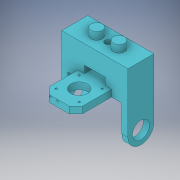
# Autodesk Inventor part: joint1_level_part_2
Saved by Autodesk Inventor 2019 (Build 230136000, 136)
## iProperties
Created: 2019-12-26
Part Number: joint1_level_part_2
Material: Пластик АБС
Document SubType Name: Modeling
Designer: Петров Иван
Density: 1.06 g/cm^3
Appearance: Серо-синий
Author: Петров Иван
Autodesk Inventor part; units mm, degrees
ref_plane "YZ Plane" through (0, 0, 0) normal (1, 0, 0) x (0, 1, 0)
ref_plane "XZ Plane" through (0, 0, 0) normal (0, 1, 0) x (-1, 0, 0)
sketch "Эскиз1" plane through (0, 0, 0) normal (1, 0, 0) x (0, 1, 0)
  line L0 (-6, -6.0208) -> (-6, 6.0208)
  arc A0 (-6, -6.0208) -> (6, -6.0208) centre (0, 0) ccw
  line L1 (6, 6.0208) -> (6, -6.0208)
  arc A1 (6, 6.0208) -> (-6, 6.0208) centre (0, 0) ccw
  circle A2 centre (0, 0) radius 17.5
  line L2 (0, 17.5) -> (80, 17.5)
  line L3 (80, 17.5) -> (80, -17.5)
  line L4 (80, -17.5) -> (0, -17.5)
  line L5 (0, -17.5) -> (0, -8.5)
  line L6 (0, 8.5) -> (0, 17.5)
  dimension "d0" = 35
  dimension "d1" = 80
  constraints: 14 end point, 6 point on circle, 3 parallel, 2 centre point, 1 coincident, 1 horizontal, 1 perpendicular, 1 vertical alignment, 2 other
  measures "d1" distance of L3.end L4.end
extrude "Выдавливание1" add sketch "Эскиз1" along normal blind 45 contours A0 L5 A2 L6 A1 L0 | A0 L1 A1 L6 A2 L5 | A2 L2 L3 L4
sketch "Эскиз2" plane through (45, 0, 0) normal (1, 0, 0) x (0, 0, -1)
  line L0 (17.5, 80) -> (-17.5, 80) projected
  line L1 (17.5, 0) -> (17.5, 80) projected
  line L2 (-17.5, 80) -> (17.5, 80)
  line L3 (17.5, 80) -> (17.5, 57)
  line L4 (17.5, 57) -> (-17.5, 57)
  line L5 (-17.5, 57) -> (-17.5, 80)
  point P0 (0, 0)
  dimension "d4" = 23
  constraints: 8 end point, 2 parallel, 1 horizontal, 1 perpendicular, 1 point on line
  measures "d4" distance of L2.end L3.end
extrude "Выдавливание2" add sketch "Эскиз2" along normal blind 22
ref_plane "РабПлоскость1" through (22.5, 0, 17.5) normal (1, 0, 0) x (0, 0, -1)
mirror "Зеркальное отражение1" about plane through (22.5, 0, 17.5) normal (1, 0, 0) of "Выдавливание2"
sketch "Эскиз3" plane through (45, 0, 0) normal (1, 0, 0) x (0, 0, -1)
  arc A0 (6.0208, -6) -> (6.0208, 6) centre (0, 0) ccw projected
  line L0 (6.0208, -6) -> (-6.0208, -6) projected
  arc A1 (-6.0208, 6) -> (-6.0208, -6) centre (0, 0) ccw projected
  line L1 (6.0208, 6) -> (-6.0208, 6) projected
  line L2 (17.5, 57) -> (-17.5, 57) projected
  line L3 (-17.5, 57) -> (-17.5, 0) projected
  arc A2 (-17.5, 0) -> (17.5, 0) centre (0, 0) ccw projected
  line L4 (17.5, 0) -> (17.5, 57) projected
sketch "Эскиз4" plane through (67, 0, 0) normal (1, 0, 0) x (0, 0, -1)
  arc A0 (6.0208, -6) -> (6.0208, 6) centre (0, 0) ccw
  line L0 (6.0208, -6) -> (-6.0208, -6)
  arc A1 (-6.0208, 6) -> (-6.0208, -6) centre (0, 0) ccw
  line L1 (6.0208, 6) -> (-6.0208, 6)
  line L2 (17.5, 37) -> (-17.5, 37)
  line L3 (-17.5, 37) -> (-17.5, 0)
  arc A2 (-17.5, 0) -> (17.5, 0) centre (0, 0) ccw
  line L4 (17.5, 0) -> (17.5, 37)
  line L5 (17.5, 0) -> (17.5, 57) projected
  line L6 (-17.5, 37) -> (17.5, 37)
  line L7 (17.5, 37) -> (17.5, 57)
  line L8 (17.5, 57) -> (-17.5, 57)
  line L9 (-17.5, 57) -> (-17.5, 37)
  constraints: 18 end point, 6 point on circle, 3 centre point, 2 parallel, 1 horizontal, 1 perpendicular
extrude "Выдавливание3" add sketch "Эскиз4" against normal blind 8
mirror "Зеркальное отражение2" about plane through (22.5, 0, 17.5) normal (1, 0, 0) of "Выдавливание3"
sketch "Эскиз5" plane through (67, 80, 17.5) normal (0, 1, 0) x (1, 0, 0)
  line L0 (-89, 35) -> (-89, 0) projected
  line L1 (-89, 35.1034) -> (-89, 0)
  line L2 (-89, 0) -> (-89, 35.1034)
  line L3 (-89, 35) -> (0, 35) projected
  line L4 (-89, 35) -> (0, 35)
  line L5 (-89, 17.5517) -> (-44.5, 17.5517)
  circle A0 centre (-44.5, 17.5517) radius 4.1
  line L6 (-44.5, 17.5517) -> (-59.5, 17.5517)
  circle A1 centre (-59.5, 17.5517) radius 7.5
  line L7 (-44.5, 17.5517) -> (-29.5, 17.5517)
  circle A2 centre (-29.5, 17.5517) radius 7.5
  point P0 (-67, 17.5)
  dimension "d9" = 8.2
  dimension "d10" = 15
  dimension "d11" = 15
  dimension "d12" = 15
  dimension "d13" = 15
  constraints: 12 end point, 3 centre point, 3 coincident, 3 collinear, 2 horizontal, 1 midpoint, 1 point on line
  measures "d9" diameter of A0
  measures "d10" distance of L6.start L6.end
  measures "d11" diameter of A1
  measures "d12" distance of L6.start L7.end
  measures "d13" diameter of A2
extrude "Выдавливание4" add sketch "Эскиз5" along normal blind 10 contours L5 A1 | L5 A1 | A2
sketch "Эскиз6" plane through (67, 80, 17.5) normal (0, 1, 0) x (1, 0, 0)
  line L0 (-89, 35) -> (-89, 0)
  line L1 (-89, 35.1034) -> (-89, 0)
  line L2 (-89, 0) -> (-89, 35.1034)
  line L3 (-89, 35) -> (0, 35)
  line L4 (-89, 35) -> (0, 35)
  line L5 (-89, 17.5517) -> (-44.5, 17.5517)
  circle A0 centre (-44.5, 17.5517) radius 4.1
  line L6 (-44.5, 17.5517) -> (-59.5, 17.5517)
  circle A1 centre (-59.5, 17.5517) radius 7.5
  line L7 (-44.5, 17.5517) -> (-29.5, 17.5517)
  circle A2 centre (-29.5, 17.5517) radius 7.5
  point P0 (-67, 17.5)
  point P1 (-67, 17.5)
  dimension "d16" = 8.2
  dimension "d17" = 15
  dimension "d18" = 15
  dimension "d19" = 15
  dimension "d20" = 15
  constraints: 16 end point, 3 centre point, 3 coincident, 3 collinear, 2 horizontal, 1 midpoint, 1 point on line
  measures "d16" diameter of A0
  measures "d17" distance of L6.start L6.end
  measures "d18" diameter of A1
  measures "d19" distance of L6.start L7.end
  measures "d20" diameter of A2
extrude "Выдавливание5" cut sketch "Эскиз6" against normal blind 35 contours A0 L7 L5 | L5 L7 A0
sketch "Эскиз7" plane through (0, 0, 17.5) normal (0, 0, 1) x (1, 0, 0)
  line L0 (18.4, 80) -> (18.4, 45) projected
  line L1 (26.6, 80) -> (26.6, 45) projected
  line L2 (0, 57) -> (0, 0) projected
  line L3 (45, 0) -> (0, 0) projected
  line L4 (45, 57) -> (45, 0) projected
  line L5 (45, 57) -> (59, 57) projected
  line L6 (67, 80) -> (67, 0) projected
  line L7 (-22, 80) -> (67, 80) projected
  line L8 (-22, 80) -> (-22, 0) projected
  line L9 (0, 57) -> (-14, 57) projected
  line L10 (18.4, 45) -> (26.6, 45) projected
  line L11 (18.4, 45) -> (8.4, 45)
  line L12 (8.4, 45) -> (8.4, 55)
  line L13 (8.4, 55) -> (36.6, 55)
  line L14 (36.6, 55) -> (36.6, 45)
  line L15 (26.6, 45) -> (36.6, 45)
  line L16 (18.4, 45) -> (26.6, 45)
  line L17 (59, 0) -> (59, 57) projected
  line L18 (67, 0) -> (59, 0) projected
  line L19 (-22, 0) -> (-14, 0) projected
  line L20 (-14, 0) -> (-14, 57) projected
  dimension "d23" = 10
  dimension "d24" = 10
  dimension "d25" = 28.2
  dimension "d26" = 10
  constraints: 12 end point, 4 perpendicular, 1 collinear, 1 horizontal, 1 point on line
  measures "d23" distance of L0.end L11.end
  measures "d24" distance of L11.end L12.end
  measures "d25" distance of L12.end L13.end
  measures "d26" distance of L1.end L14.end
extrude "Выдавливание6" cut sketch "Эскиз7" against normal blind 84.5 contours L13 L1 L10 L0 | L0 L11 L12 L13 | L13 L14 L15 L1
sketch "Эскиз8" plane through (0, 0, 17.5) normal (0, 0, 1) x (1, 0, 0)
  line L0 (8.4, 45) -> (36.6, 45) projected
  line L1 (8.4, 45) -> (0, 45)
  line L2 (0, 45) -> (0, 36)
  line L3 (0, 0) -> (0, 57) projected
  line L4 (45, -17.5) -> (45, 0) projected
  line L5 (0, 36) -> (45, 36)
  line L6 (45, 36) -> (45, -17.5)
  line L7 (45, -17.5) -> (0, -17.5)
  line L8 (0, -17.5) -> (0, 36)
  dimension "d29" = 9
  constraints: 12 end point, 2 horizontal, 2 parallel, 1 perpendicular, 1 point on line
  measures "d29" distance of L1.end L2.end
extrude "Выдавливание7" cut sketch "Эскиз8" against normal blind 85.25
sketch "Эскиз9" plane through (67, 0, 0) normal (1, 0, 0) x (0, 0, -1)
  circle A0 centre (0, 0) radius 11.4
  dimension "d32" = 22.8
  constraints: 1 centre point, 1 coincident
  measures "d32" diameter of A0
extrude "Выдавливание8" cut sketch "Эскиз9" against normal blind 144.5
sketch "Эскиз10" plane through (-22, 80, 17.5) normal (0, 0, 1) x (1, 0, 0)
  line L0 (22, -23) -> (22, -44) projected
  line L1 (67, -23) -> (67, -44) projected
  line L2 (22, -44) -> (67, -44)
  line L3 (67, -44) -> (67, -35)
  line L4 (67, -35) -> (22, -35)
  line L5 (22, -35) -> (22, -44)
  point P0 (22, -80)
  dimension "d35" = 9
  constraints: 8 end point, 2 parallel, 1 horizontal, 1 perpendicular, 1 point on line
  measures "d35" distance of L3.end L2.end
extrude "Выдавливание9" add sketch "Эскиз10" along normal blind 45
sketch "Эскиз11" plane through (67, 45, 17.5) normal (0, 1, 0) x (1, 0, 0)
  line L0 (-67, 0) -> (-67, 35) projected
  line L1 (-67, 0) -> (-44.5, 0)
  line L2 (-67, 0) -> (-58.6, 0) projected
  line L3 (-22, -45) -> (-67, -45) projected
  line L4 (-44.5, -45) -> (-44.5, -21)
  line L5 (-27, -42) -> (-23.5, -38.5)
  line L6 (-23.5, -38.5) -> (-23.5, -3.5)
  line L7 (-23.5, -3.5) -> (-27, 0)
  line L8 (-27, 0) -> (-62, 0)
  line L9 (-62, 0) -> (-65.5, -3.5)
  line L10 (-65.5, -3.5) -> (-65.5, -38.5)
  line L11 (-65.5, -38.5) -> (-62, -42)
  line L12 (-62, -42) -> (-27, -42)
  circle A0 centre (-44.5, -21) radius 11.3
  circle A1 centre (-29, -5.5) radius 1.25
  circle A2 centre (-60, -5.5) radius 1.25
  circle A3 centre (-60, -36.5) radius 1.25
  circle A4 centre (-29, -36.5) radius 1.25
  line L13 (-52.5, -48) -> (-50.5, -48)
  line L14 (-50.5, -41.8) -> (-50.5, -48)
  line L15 (-57.9172, -41.8) -> (-50.5, -41.8)
  line L16 (-65.3, -34.4172) -> (-57.9172, -41.8)
  line L17 (-65.3, -7.5828) -> (-65.3, -34.4172)
  line L18 (-57.9172, -0.2) -> (-65.3, -7.5828)
  line L19 (-31.0828, -0.2) -> (-57.9172, -0.2)
  line L20 (-23.7, -7.5828) -> (-31.0828, -0.2)
  line L21 (-23.7, -34.4172) -> (-23.7, -7.5828)
  line L22 (-31.0828, -41.8) -> (-23.7, -34.4172)
  line L23 (-38.5, -41.8) -> (-31.0828, -41.8)
  line L24 (-38.5, -41.8) -> (-38.5, -48)
  line L25 (-38.5, -48) -> (-36.5, -48)
  line L26 (-36.5, -48) -> (-36.5, -42)
  line L27 (-36.5, -42) -> (-27, -42)
  line L28 (-27, -42) -> (-23.5, -38.5)
  line L29 (-23.5, -38.5) -> (-23.5, -3.5)
  line L30 (-23.5, -3.5) -> (-27, 0)
  line L31 (-27, 0) -> (-62, 0)
  line L32 (-62, 0) -> (-65.5, -3.5)
  line L33 (-65.5, -3.5) -> (-65.5, -38.5)
  line L34 (-65.5, -38.5) -> (-62, -42)
  line L35 (-62, -42) -> (-52.5, -42)
  line L36 (-52.5, -42) -> (-52.5, -48)
  point P0 (-67, 17.5)
  dimension "d38" = 22.5
  dimension "d39" = 24
  constraints: 68 end point, 5 centre point, 1 collinear, 1 midpoint, 1 vertical
  measures "d38" distance of L0.start L1.end
  measures "d39" distance of L4.start L4.end
extrude "Выдавливание10" cut sketch "Эскиз11" against normal blind 45 contours A0 | A1 | A2 | A3 | A4
chamfer "Фаска1" distance 2 angle 45 4 edges at (5.75, 36, 54) (5.75, 36, 23) (36.75, 36, 23) (36.75, 36, 54)
chamfer "Фаска2" distance 6 angle 45 2 edges at (0, 40.5, 62.5) (45, 40.5, 62.5)
sketch "Эскиз13" plane through (-22, 80, 17.5) normal (0, 0, 1) x (1, 0, 0)
  line L0 (81, -80) -> (81, -23) projected
  line L1 (22, -23) -> (8, -23) projected
  line L2 (81, -44) -> (8, -44)
  line L3 (8, -44) -> (8, -23)
  line L4 (8, -23) -> (81, -23)
  line L5 (81, -23) -> (81, -44)
  line L6 (61, -44) -> (67, -44) projected
  line L7 (22, -35) -> (30.4, -35) projected
  line L8 (30.4, -25) -> (58.6, -25) projected
  line L9 (30.4, -35) -> (58.6, -35)
  line L10 (58.6, -35) -> (58.6, -25)
  line L11 (58.6, -25) -> (30.4, -25)
  line L12 (30.4, -25) -> (30.4, -35)
  point P0 (22, -80)
  dimension "d51" = 0
  constraints: 16 end point, 4 parallel, 2 horizontal, 2 perpendicular, 1 point on line
  measures "d51" distance between parallel lines of L6 L2
extrude "Выдавливание12" add sketch "Эскиз13" against normal up to surface (35 mm away)
sketch "Эскиз14" plane through (-22, 80, 62.5) normal (0, 0, 1) x (1, 0, 0)
  line L0 (27.8074, -44.5836) -> (28.32, -44.5836)
  line L1 (28.32, -44.5836) -> (28.4117, -43.1496)
  arc A0 (32.6031, -43.1496) -> (28.4117, -43.1496) centre (30.5074, -43.2836) ccw
  line L2 (32.6031, -43.1496) -> (32.6948, -44.5836)
  line L3 (32.6948, -44.5836) -> (36.9831, -44.5836)
  arc A1 (36.9831, -44.5836) -> (37.0538, -44.5543) centre (36.9831, -44.4836) ccw
  line L4 (37.0538, -44.5543) -> (37.3781, -44.23)
  arc A2 (37.7316, -44.0836) -> (37.3781, -44.23) centre (37.7316, -44.5836) ccw
  line L5 (37.7316, -44.0836) -> (47.4074, -44.0836)
  arc A3 (47.4074, -44.0836) -> (47.5074, -43.9836) centre (47.4074, -43.9836) ccw
  line L6 (47.5074, -43.9836) -> (47.5074, -34.8336)
  arc A4 (47.5074, -34.8336) -> (47.4074, -34.7336) centre (47.4074, -34.8336) ccw
  line L7 (47.4074, -34.7336) -> (44.4816, -34.7336)
  arc A5 (44.1281, -34.5871) -> (44.4816, -34.7336) centre (44.4816, -34.2336) ccw
  line L8 (44.1281, -34.5871) -> (43.8038, -34.2629)
  arc A6 (43.8038, -34.2629) -> (43.7331, -34.2336) centre (43.7331, -34.3336) ccw
  line L9 (43.7331, -34.2336) -> (40.9816, -34.2336)
  arc A7 (40.9816, -34.2336) -> (40.9109, -34.2629) centre (40.9816, -34.3336) ccw
  line L10 (40.9109, -34.2629) -> (40.5867, -34.5871)
  arc A8 (40.2331, -34.7336) -> (40.5867, -34.5871) centre (40.2331, -34.2336) ccw
  line L11 (40.2331, -34.7336) -> (34.9816, -34.7336)
  arc A9 (34.6281, -34.5871) -> (34.9816, -34.7336) centre (34.9816, -34.2336) ccw
  line L12 (34.6281, -34.5871) -> (34.3038, -34.2629)
  arc A10 (34.3038, -34.2629) -> (34.2331, -34.2336) centre (34.2331, -34.3336) ccw
  line L13 (34.2331, -34.2336) -> (31.4816, -34.2336)
  arc A11 (31.4816, -34.2336) -> (31.4109, -34.2629) centre (31.4816, -34.3336) ccw
  line L14 (31.4109, -34.2629) -> (31.0867, -34.5871)
  arc A12 (30.7331, -34.7336) -> (31.0867, -34.5871) centre (30.7331, -34.2336) ccw
  line L15 (30.7331, -34.7336) -> (27.8074, -34.7336)
  arc A13 (27.8074, -34.7336) -> (27.7074, -34.8336) centre (27.8074, -34.8336) ccw
  line L16 (27.7074, -34.8336) -> (27.7074, -44.4836)
  arc A14 (27.7074, -44.4836) -> (27.8074, -44.5836) centre (27.8074, -44.4836) ccw
  circle A15 centre (32.8574, -36.7836) radius 1.25
  circle A16 centre (42.3574, -36.7836) radius 1.25
  line L17 (43.5307, -39.0336) -> (42.914, -40.3336)
  line L18 (42.914, -40.3336) -> (42.8974, -40.3336)
  line L19 (42.8974, -40.3336) -> (42.2974, -39.0336)
  line L20 (42.2974, -39.0336) -> (42.4242, -39.0336)
  line L21 (42.4242, -39.0336) -> (42.6164, -39.4502)
  line L22 (42.6164, -39.4502) -> (43.2057, -39.4502)
  line L23 (43.2057, -39.4502) -> (43.4034, -39.0336)
  line L24 (43.4034, -39.0336) -> (43.5307, -39.0336)
  spline S0 degree 3 poles (40.7107, -39.97) (40.711, -39.9789) (40.7114, -39.9964) (40.7155, -40.022) (40.7217, -40.0467) (40.7306, -40.0706) (40.7424, -40.0934) (40.7567, -40.1152) (40.7731, -40.1363) (40.7922, -40.156) (40.8132, -40.1741) (40.8353, -40.1901) (40.8587, -40.2035) (40.8833, -40.2145) (40.909, -40.2231) (40.9359, -40.2291) (40.9639, -40.2328) (40.983, -40.2333) (40.9927, -40.2336) knots 0 0 0 0 0.061965 0.122122 0.180988 0.239933 0.299906 0.359989 0.421776 0.486576 0.551535 0.615018 0.677259 0.73973 0.80305 0.866495 0.931973 1 1 1 1
  spline S1 degree 3 poles (40.9927, -40.2336) (41.0029, -40.2333) (41.0229, -40.2328) (41.0522, -40.2291) (41.0802, -40.2228) (41.1068, -40.2142) (41.1323, -40.2033) (41.1564, -40.1897) (41.1791, -40.1734) (41.2004, -40.155) (41.22, -40.1344) (41.2373, -40.1115) (41.2523, -40.0867) (41.2655, -40.06) (41.2762, -40.0312) (41.2843, -40.0004) (41.2908, -39.9677) (41.2929, -39.9451) (41.294, -39.9336) knots 0 0 0 0 0.064439 0.126547 0.186887 0.245878 0.304041 0.362191 0.420976 0.48066 0.5406 0.600689 0.661936 0.724443 0.789038 0.856314 0.926352 1 1 1 1
  line L25 (41.294, -39.9336) -> (41.4107, -39.9336)
  spline S2 degree 3 poles (41.4107, -39.9336) (41.41, -39.949) (41.4085, -39.9794) (41.4015, -40.0238) (41.3915, -40.0661) (41.3773, -40.1062) (41.3597, -40.1443) (41.3387, -40.1803) (41.3137, -40.2141) (41.2854, -40.2454) (41.2547, -40.2741) (41.2215, -40.2988) (41.1866, -40.3197) (41.1502, -40.3372) (41.1118, -40.3504) (41.0717, -40.3601) (41.0298, -40.366) (41.0013, -40.3666) (40.9868, -40.3669) knots 0 0 0 0 0.068791 0.135103 0.198979 0.261904 0.323495 0.385195 0.446969 0.509765 0.572251 0.633405 0.693251 0.752583 0.812579 0.873275 0.93555 1 1 1 1
  spline S3 degree 3 poles (40.9868, -40.3669) (40.9725, -40.3666) (40.9445, -40.3659) (40.9036, -40.3603) (40.8647, -40.3515) (40.8278, -40.3391) (40.7933, -40.3225) (40.7608, -40.3025) (40.73, -40.2794) (40.7023, -40.2522) (40.6769, -40.2231) (40.6549, -40.1921) (40.6361, -40.1601) (40.6204, -40.1268) (40.6089, -40.0919) (40.6001, -40.056) (40.5952, -40.0186) (40.5944, -39.9933) (40.594, -39.9804) knots 0 0 0 0 0.069475 0.136517 0.200789 0.26383 0.325735 0.387291 0.449509 0.512968 0.576275 0.63758 0.697903 0.757172 0.816599 0.876653 0.93729 1 1 1 1
  spline S4 degree 3 poles (40.594, -39.9804) (40.5947, -39.9623) (40.5959, -39.9264) (40.6066, -39.8737) (40.6232, -39.8226) (40.6433, -39.7815) (40.6635, -39.7483) (40.6818, -39.721) (40.7031, -39.6916) (40.7279, -39.6603) (40.7556, -39.6266) (40.7864, -39.5908) (40.8206, -39.5531) (40.8446, -39.5274) (40.8571, -39.514) knots 0 0 0 0 0.098702 0.195672 0.292422 0.391343 0.444462 0.504229 0.570352 0.642546 0.722288 0.807921 0.90047 1 1 1 1
  line L26 (40.8571, -39.514) -> (41.1823, -39.1669)
  line L27 (41.1823, -39.1669) -> (40.5774, -39.1669)
  line L28 (40.5774, -39.1669) -> (40.5774, -39.0336)
  line L29 (40.5774, -39.0336) -> (41.4607, -39.0336)
  line L30 (41.4607, -39.0336) -> (40.9565, -39.5716)
  spline S5 degree 3 poles (40.9565, -39.5716) (40.9443, -39.5844) (40.9207, -39.609) (40.8873, -39.6449) (40.8574, -39.6783) (40.8306, -39.709) (40.8077, -39.7374) (40.7873, -39.7628) (40.771, -39.7861) (40.7532, -39.8131) (40.7361, -39.8461) (40.7213, -39.8864) (40.7123, -39.9279) (40.7113, -39.9559) (40.7107, -39.97) knots 0 0 0 0 0.110803 0.212829 0.306101 0.390647 0.466924 0.534481 0.593587 0.644557 0.7362 0.825024 0.911986 1 1 1 1
  line L31 (40.2007, -39.6836) -> (40.0674, -40.3336)
  line L32 (40.0674, -40.3336) -> (39.534, -40.3336)
  line L33 (39.534, -40.3336) -> (39.534, -40.2002)
  line L34 (39.534, -40.2002) -> (39.9762, -40.2002)
  line L35 (39.9762, -40.2002) -> (40.0463, -39.8583)
  spline S6 degree 3 poles (40.0463, -39.8583) (40.0325, -39.8621) (40.0059, -39.8695) (39.9665, -39.8776) (39.9291, -39.8826) (39.9049, -39.8832) (39.8932, -39.8836) knots 0 0 0 0 0.275068 0.532901 0.773973 1 1 1 1
  spline S7 degree 3 poles (39.8932, -39.8836) (39.8786, -39.8833) (39.8501, -39.8826) (39.8083, -39.8767) (39.7685, -39.8674) (39.7306, -39.8543) (39.6946, -39.8376) (39.6609, -39.8168) (39.6289, -39.7925) (39.5992, -39.7645) (39.5722, -39.7337) (39.5486, -39.7006) (39.5284, -39.6655) (39.5123, -39.628) (39.4993, -39.5887) (39.4907, -39.547) (39.485, -39.5033) (39.4844, -39.4735) (39.484, -39.4583) knots 0 0 0 0 0.065808 0.129394 0.190894 0.251281 0.310815 0.370371 0.430768 0.492881 0.555104 0.616067 0.677256 0.73826 0.800762 0.864778 0.931045 1 1 1 1
  spline S8 degree 3 poles (39.484, -39.4583) (39.4843, -39.4477) (39.4848, -39.4267) (39.4873, -39.3954) (39.4921, -39.3648) (39.4985, -39.3349) (39.5069, -39.3057) (39.517, -39.2771) (39.5295, -39.2493) (39.5431, -39.2221) (39.5584, -39.196) (39.5754, -39.1716) (39.5933, -39.1485) (39.6127, -39.1271) (39.6335, -39.1073) (39.6557, -39.0891) (39.679, -39.0722) (39.7038, -39.0573) (39.7294, -39.0436) (39.7564, -39.0323) (39.7841, -39.0222) (39.8128, -39.0142) (39.8426, -39.0079) (39.8734, -39.0036) (39.9051, -39.0005) (39.9266, -39.0003) (39.9374, -39.0002) knots 0 0 0 0 0.044014 0.087434 0.130118 0.172554 0.214555 0.256298 0.298438 0.340849 0.382715 0.423924 0.464246 0.504074 0.543862 0.583567 0.623094 0.663229 0.703551 0.743938 0.784541 0.82575 0.867757 0.910745 0.954914 1 1 1 1
  spline S9 degree 3 poles (39.9374, -39.0002) (39.9504, -39.0005) (39.9759, -39.001) (40.0132, -39.0063) (40.0491, -39.0138) (40.0834, -39.0252) (40.1162, -39.0395) (40.1472, -39.0575) (40.1771, -39.0779) (40.2048, -39.102) (40.2305, -39.1284) (40.2535, -39.1569) (40.2739, -39.1873) (40.2916, -39.2196) (40.3066, -39.2537) (40.3184, -39.2898) (40.328, -39.3276) (40.332, -39.3537) (40.334, -39.3669) knots 0 0 0 0 0.065421 0.128708 0.190236 0.250724 0.310637 0.370766 0.431615 0.493523 0.555883 0.617342 0.678668 0.740711 0.802985 0.866803 0.932347 1 1 1 1
  line L36 (40.334, -39.3669) -> (40.2174, -39.3669)
  spline S10 degree 3 poles (40.2174, -39.3669) (40.2145, -39.3545) (40.209, -39.3307) (40.1969, -39.2972) (40.1821, -39.2674) (40.1645, -39.2408) (40.1435, -39.2176) (40.1195, -39.1969) (40.0926, -39.1783) (40.0628, -39.1628) (40.0313, -39.1495) (39.9983, -39.1407) (39.9647, -39.1345) (39.9421, -39.1339) (39.9307, -39.1336) knots 0 0 0 0 0.094687 0.181994 0.264377 0.34218 0.418618 0.496509 0.577369 0.661511 0.746733 0.831258 0.915206 1 1 1 1
  spline S11 degree 3 poles (39.9307, -39.1336) (39.9195, -39.1339) (39.8976, -39.1345) (39.8654, -39.1391) (39.8343, -39.1462) (39.8045, -39.1569) (39.7757, -39.1698) (39.7486, -39.1864) (39.7222, -39.2055) (39.6975, -39.2274) (39.6749, -39.2516) (39.655, -39.2774) (39.6384, -39.3049) (39.6243, -39.3337) (39.6137, -39.364) (39.6061, -39.3958) (39.6016, -39.429) (39.601, -39.4517) (39.6007, -39.4633) knots 0 0 0 0 0.064207 0.126425 0.18768 0.248216 0.308305 0.369661 0.431699 0.495947 0.559758 0.622295 0.683911 0.745092 0.80674 0.869087 0.93329 1 1 1 1
  spline S12 degree 3 poles (39.6007, -39.4633) (39.601, -39.4737) (39.6014, -39.4941) (39.6054, -39.524) (39.6122, -39.5522) (39.6216, -39.579) (39.6336, -39.6043) (39.6482, -39.6283) (39.6658, -39.6504) (39.6859, -39.6709) (39.7079, -39.6898) (39.7322, -39.7059) (39.7583, -39.7194) (39.7859, -39.7311) (39.8156, -39.7395) (39.8468, -39.7458) (39.88, -39.7495) (39.9026, -39.75) (39.9143, -39.7502) knots 0 0 0 0 0.065351 0.127916 0.18836 0.247216 0.30563 0.36377 0.422661 0.482687 0.5433 0.604118 0.664965 0.727413 0.791468 0.858055 0.927037 1 1 1 1
  spline S13 degree 3 poles (39.9143, -39.7502) (39.9243, -39.75) (39.9451, -39.7496) (39.9771, -39.7463) (40.0106, -39.741) (40.0456, -39.7337) (40.0823, -39.7242) (40.1204, -39.7128) (40.1602, -39.6992) (40.1869, -39.6889) (40.2007, -39.6836) knots 0 0 0 0 0.102203 0.211023 0.3251 0.446502 0.573788 0.708901 0.850358 1 1 1 1
  line L37 (36.754, -39.0336) -> (36.1374, -40.3336)
  line L38 (36.1374, -40.3336) -> (36.1207, -40.3336)
  line L39 (36.1207, -40.3336) -> (35.5207, -39.0336)
  line L40 (35.5207, -39.0336) -> (35.6475, -39.0336)
  line L41 (35.6475, -39.0336) -> (35.8397, -39.4502)
  line L42 (35.8397, -39.4502) -> (36.429, -39.4502)
  line L43 (36.429, -39.4502) -> (36.6267, -39.0336)
  line L44 (36.6267, -39.0336) -> (36.754, -39.0336)
  spline S14 degree 3 poles (35.244, -39.6911) (35.2435, -39.7145) (35.2423, -39.7605) (35.2327, -39.828) (35.2171, -39.8927) (35.1951, -39.9544) (35.1671, -40.0135) (35.1326, -40.0696) (35.0918, -40.1229) (35.0452, -40.1727) (34.9941, -40.2182) (34.9394, -40.2582) (34.8812, -40.2915) (34.8201, -40.3194) (34.7556, -40.3408) (34.688, -40.3558) (34.6173, -40.3651) (34.5691, -40.3663) (34.5446, -40.3669) knots 0 0 0 0 0.064558 0.127014 0.187955 0.248014 0.307748 0.368235 0.42947 0.492743 0.556258 0.618217 0.679655 0.741246 0.803415 0.866815 0.932328 1 1 1 1
  spline S15 degree 3 poles (34.5446, -40.3669) (34.5296, -40.3667) (34.5001, -40.3664) (34.4563, -40.3629) (34.4137, -40.3571) (34.3723, -40.3493) (34.3318, -40.3396) (34.2925, -40.3269) (34.2542, -40.3124) (34.2171, -40.2957) (34.1815, -40.2769) (34.1473, -40.2564) (34.1148, -40.234) (34.0838, -40.21) (34.0548, -40.1838) (34.0269, -40.1562) (34.0012, -40.1265) (33.9853, -40.1055) (33.9774, -40.095) knots 0 0 0 0 0.068548 0.135683 0.201215 0.265682 0.329267 0.392395 0.45507 0.517127 0.57879 0.63974 0.700192 0.759806 0.819628 0.879355 0.939512 1 1 1 1
  line L45 (33.9774, -40.095) -> (34.0795, -40.0169)
  spline S16 degree 3 poles (34.0795, -40.0169) (34.0867, -40.0256) (34.1012, -40.0428) (34.1245, -40.067) (34.1487, -40.0897) (34.174, -40.111) (34.2006, -40.1301) (34.2281, -40.148) (34.2567, -40.1641) (34.2964, -40.1836) (34.3483, -40.2039) (34.4135, -40.2209) (34.4817, -40.2318) (34.5282, -40.233) (34.5519, -40.2336) knots 0 0 0 0 0.063163 0.125475 0.187121 0.248294 0.309295 0.36985 0.430973 0.492456 0.616148 0.740844 0.868183 1 1 1 1
  spline S17 degree 3 poles (34.5519, -40.2336) (34.5649, -40.2334) (34.5908, -40.2331) (34.6293, -40.2292) (34.6671, -40.2236) (34.7041, -40.2154) (34.7404, -40.205) (34.7761, -40.1926) (34.8107, -40.1773) (34.8447, -40.1603) (34.8773, -40.1411) (34.9082, -40.1202) (34.9372, -40.0978) (34.9643, -40.0738) (34.9896, -40.0483) (35.0129, -40.021) (35.0342, -39.9921) (35.0538, -39.9619) (35.0713, -39.9305) (35.086, -39.8978) (35.099, -39.8643) (35.1093, -39.8297) (35.1174, -39.7942) (35.123, -39.7577) (35.1269, -39.7204) (35.1272, -39.695) (35.1274, -39.6823) knots 0 0 0 0 0.043955 0.087502 0.130463 0.172752 0.215403 0.25765 0.300153 0.343121 0.385925 0.427686 0.468818 0.509492 0.549883 0.58998 0.630405 0.670869 0.711384 0.751627 0.791776 0.832459 0.873319 0.914543 0.956924 1 1 1 1
  spline S18 degree 3 poles (35.1274, -39.6823) (35.1269, -39.6631) (35.126, -39.6253) (35.1178, -39.5701) (35.1054, -39.5171) (35.0867, -39.4668) (35.0637, -39.4186) (35.0346, -39.3732) (35.001, -39.33) (34.9623, -39.2899) (34.9198, -39.2533) (34.8742, -39.2211) (34.8256, -39.1942) (34.7746, -39.1719) (34.7207, -39.1547) (34.6641, -39.1426) (34.6049, -39.1347) (34.5644, -39.134) (34.5438, -39.1336) knots 0 0 0 0 0.064323 0.12629 0.186726 0.246146 0.305576 0.365429 0.426326 0.48884 0.551725 0.613919 0.675484 0.737334 0.800229 0.864502 0.931041 1 1 1 1
  spline S19 degree 3 poles (34.5438, -39.1336) (34.5211, -39.1342) (34.4764, -39.1354) (34.4109, -39.1459) (34.3482, -39.1628) (34.2883, -39.1866) (34.2313, -39.2174) (34.1773, -39.2548) (34.126, -39.2991) (34.0952, -39.333) (34.0795, -39.3502) knots 0 0 0 0 0.128515 0.252949 0.374755 0.49594 0.617181 0.740909 0.867811 1 1 1 1
  line L46 (34.0795, -39.3502) -> (33.9774, -39.2729)
  spline S20 degree 3 poles (33.9774, -39.2729) (33.9856, -39.2623) (34.002, -39.2411) (34.0285, -39.2113) (34.0565, -39.1833) (34.0861, -39.1572) (34.1169, -39.1327) (34.1497, -39.1103) (34.1838, -39.0897) (34.2192, -39.0709) (34.2559, -39.0542) (34.2938, -39.04) (34.3327, -39.0277) (34.3727, -39.0175) (34.4138, -39.0096) (34.4559, -39.0043) (34.4991, -39.0007) (34.5282, -39.0004) (34.543, -39.0002) knots 0 0 0 0 0.061674 0.123053 0.183475 0.243727 0.304279 0.364863 0.425946 0.487391 0.54922 0.611144 0.673529 0.736961 0.800785 0.866013 0.932101 1 1 1 1
  spline S21 degree 3 poles (34.543, -39.0002) (34.557, -39.0003) (34.5846, -39.0005) (34.6255, -39.0036) (34.6652, -39.0079) (34.7037, -39.0143) (34.7413, -39.0219) (34.7775, -39.032) (34.8128, -39.0433) (34.847, -39.0567) (34.88, -39.0717) (34.9119, -39.0887) (34.9426, -39.1075) (34.9724, -39.1278) (35.0009, -39.1501) (35.0282, -39.1741) (35.0546, -39.1998) (35.071, -39.2183) (35.0792, -39.2276) knots 0 0 0 0 0.069663 0.13775 0.203917 0.26878 0.332414 0.394754 0.45618 0.516996 0.577396 0.637198 0.696999 0.756756 0.816554 0.876948 0.938132 1 1 1 1
  spline S22 degree 3 poles (35.0792, -39.2276) (35.0924, -39.2438) (35.1185, -39.2759) (35.152, -39.328) (35.1807, -39.3824) (35.2038, -39.4394) (35.2219, -39.4988) (35.2345, -39.5608) (35.2426, -39.6251) (35.2436, -39.6689) (35.244, -39.6911) knots 0 0 0 0 0.124329 0.247156 0.36878 0.490734 0.613614 0.738958 0.867311 1 1 1 1
  line L47 (32.1714, -40.2836) -> (32.3842, -40.2836)
  line L48 (32.5718, -39.1836) -> (32.1714, -40.2836)
  line L49 (32.0718, -39.1836) -> (32.5718, -39.1836)
  line L50 (31.6714, -40.2836) -> (32.0718, -39.1836)
  line L51 (31.4585, -40.2836) -> (31.6714, -40.2836)
  line L52 (31.8589, -39.1836) -> (31.4585, -40.2836)
  line L53 (31.6589, -39.1836) -> (31.8589, -39.1836)
  line L54 (31.7317, -38.9836) -> (31.6589, -39.1836)
  line L55 (32.8574, -38.9836) -> (31.7317, -38.9836)
  line L56 (32.3842, -40.2836) -> (32.8574, -38.9836)
  line L57 (37.5474, -39.0336) -> (37.564, -39.0336)
  line L58 (37.564, -39.0336) -> (38.114, -40.3336)
  line L59 (38.114, -40.3336) -> (37.989, -40.3336)
  line L60 (37.989, -40.3336) -> (37.5557, -39.3091)
  line L61 (37.5557, -39.3091) -> (37.1224, -40.3336)
  line L62 (37.1224, -40.3336) -> (36.9974, -40.3336)
  line L63 (36.9974, -40.3336) -> (37.5474, -39.0336)
  spline S23 degree 3 poles (38.3574, -39.683) (38.3576, -39.6632) (38.3581, -39.6244) (38.3605, -39.5678) (38.3654, -39.5143) (38.3714, -39.4638) (38.3797, -39.4167) (38.39, -39.3725) (38.4014, -39.3313) (38.4154, -39.2934) (38.4308, -39.2581) (38.4475, -39.2252) (38.4654, -39.1943) (38.485, -39.1657) (38.5058, -39.1392) (38.5284, -39.1152) (38.552, -39.0932) (38.577, -39.0737) (38.6032, -39.0566) (38.6299, -39.0412) (38.6577, -39.0289) (38.6859, -39.0183) (38.7149, -39.0102) (38.7447, -39.0046) (38.7752, -39.0007) (38.7957, -39.0004) (38.8061, -39.0002) knots 0 0 0 0 0.065063 0.126773 0.185516 0.240765 0.29298 0.34225 0.388919 0.432776 0.474628 0.514775 0.553606 0.591426 0.628028 0.663804 0.698984 0.733591 0.767628 0.801208 0.834264 0.866981 0.89972 0.932702 0.966176 1 1 1 1
  spline S24 degree 3 poles (38.8061, -39.0002) (38.8163, -39.0004) (38.8365, -39.0007) (38.8665, -39.0043) (38.8956, -39.01) (38.9239, -39.0179) (38.9517, -39.0277) (38.9784, -39.0403) (39.0046, -39.055) (39.0299, -39.0716) (39.0541, -39.0907) (39.0771, -39.1117) (39.0985, -39.1354) (39.1185, -39.1612) (39.1374, -39.1889) (39.1548, -39.219) (39.1709, -39.2512) (39.1856, -39.2859) (39.1987, -39.3235) (39.2102, -39.3644) (39.2193, -39.409) (39.2271, -39.4569) (39.2334, -39.5085) (39.2377, -39.5635) (39.2404, -39.6222) (39.2406, -39.6624) (39.2407, -39.683) knots 0 0 0 0 0.033787 0.066622 0.099285 0.131361 0.163585 0.196104 0.228902 0.262158 0.295991 0.330218 0.36506 0.400951 0.43762 0.475708 0.515381 0.556414 0.599765 0.646424 0.696431 0.749782 0.806573 0.867436 0.931887 1 1 1 1
  spline S25 degree 3 poles (39.2407, -39.683) (39.2406, -39.7039) (39.2404, -39.7444) (39.2377, -39.8033) (39.2334, -39.8587) (39.2274, -39.9103) (39.2201, -39.9584) (39.2103, -40.0027) (39.1993, -40.0434) (39.1864, -40.0807) (39.1719, -40.1151) (39.1562, -40.1472) (39.1385, -40.177) (39.1199, -40.2049) (39.0997, -40.2305) (39.0785, -40.2541) (39.0553, -40.2753) (39.031, -40.2945) (39.0053, -40.3114) (38.9791, -40.3263) (38.9521, -40.339) (38.9242, -40.3489) (38.8957, -40.3572) (38.8665, -40.3628) (38.8366, -40.3664) (38.8163, -40.3667) (38.8061, -40.3669) knots 0 0 0 0 0.068595 0.133246 0.194313 0.251279 0.304513 0.354235 0.400481 0.443411 0.484015 0.523252 0.561042 0.5979 0.633518 0.668314 0.702496 0.736685 0.770293 0.803437 0.835913 0.86846 0.900847 0.933467 0.966258 1 1 1 1
  spline S26 degree 3 poles (38.8061, -40.3669) (38.7957, -40.3667) (38.7752, -40.3664) (38.7448, -40.3629) (38.7151, -40.3572) (38.6862, -40.349) (38.6579, -40.3389) (38.6305, -40.3262) (38.6037, -40.3115) (38.5779, -40.2942) (38.5529, -40.2749) (38.5294, -40.2531) (38.5072, -40.2289) (38.4862, -40.2028) (38.4668, -40.1741) (38.4484, -40.1433) (38.4319, -40.11) (38.4161, -40.0746) (38.4024, -40.0363) (38.39, -39.9951) (38.38, -39.9507) (38.3717, -39.9033) (38.3653, -39.8526) (38.3606, -39.7988) (38.3581, -39.7419) (38.3576, -39.703) (38.3574, -39.683) knots 0 0 0 0 0.033788 0.067194 0.099862 0.132567 0.165151 0.197913 0.231319 0.265083 0.299255 0.334399 0.369943 0.406284 0.444064 0.482998 0.523354 0.565537 0.609613 0.656391 0.705885 0.758325 0.813832 0.872795 0.934722 1 1 1 1
  line L64 (44.5074, -39.6836) -> (44.374, -40.3336)
  line L65 (44.374, -40.3336) -> (43.8407, -40.3336)
  line L66 (43.8407, -40.3336) -> (43.8407, -40.2002)
  line L67 (43.8407, -40.2002) -> (44.2829, -40.2002)
  line L68 (44.2829, -40.2002) -> (44.353, -39.8583)
  spline S27 degree 3 poles (44.353, -39.8583) (44.3392, -39.8621) (44.3125, -39.8695) (44.2732, -39.8776) (44.2358, -39.8826) (44.2116, -39.8832) (44.1998, -39.8836) knots 0 0 0 0 0.275068 0.532901 0.773973 1 1 1 1
  spline S28 degree 3 poles (44.1998, -39.8836) (44.1853, -39.8833) (44.1568, -39.8826) (44.115, -39.8767) (44.0751, -39.8674) (44.0373, -39.8543) (44.0013, -39.8376) (43.9675, -39.8168) (43.9355, -39.7925) (43.9058, -39.7645) (43.8789, -39.7337) (43.8552, -39.7006) (43.8351, -39.6655) (43.8189, -39.628) (43.806, -39.5887) (43.7974, -39.547) (43.7917, -39.5033) (43.791, -39.4735) (43.7907, -39.4583) knots 0 0 0 0 0.065808 0.129394 0.190894 0.251281 0.310815 0.370371 0.430768 0.492881 0.555104 0.616067 0.677256 0.73826 0.800762 0.864778 0.931045 1 1 1 1
  spline S29 degree 3 poles (43.7907, -39.4583) (43.791, -39.4477) (43.7915, -39.4267) (43.7939, -39.3954) (43.7988, -39.3648) (43.8052, -39.3349) (43.8136, -39.3057) (43.8237, -39.2771) (43.8361, -39.2493) (43.8497, -39.2221) (43.865, -39.196) (43.882, -39.1716) (43.9, -39.1485) (43.9193, -39.1271) (43.9402, -39.1073) (43.9624, -39.0891) (43.9857, -39.0722) (44.0104, -39.0573) (44.0361, -39.0436) (44.0631, -39.0323) (44.0907, -39.0222) (44.1195, -39.0142) (44.1492, -39.0079) (44.18, -39.0036) (44.2117, -39.0005) (44.2332, -39.0003) (44.2441, -39.0002) knots 0 0 0 0 0.044014 0.087434 0.130118 0.172554 0.214555 0.256298 0.298438 0.340849 0.382715 0.423924 0.464246 0.504074 0.543862 0.583567 0.623094 0.663229 0.703551 0.743938 0.784541 0.82575 0.867757 0.910745 0.954914 1 1 1 1
  spline S30 degree 3 poles (44.2441, -39.0002) (44.2571, -39.0005) (44.2825, -39.001) (44.3199, -39.0063) (44.3558, -39.0138) (44.39, -39.0252) (44.4228, -39.0395) (44.4538, -39.0575) (44.4838, -39.0779) (44.5114, -39.102) (44.5371, -39.1284) (44.5601, -39.1569) (44.5806, -39.1873) (44.5982, -39.2196) (44.6133, -39.2537) (44.6251, -39.2898) (44.6346, -39.3276) (44.6387, -39.3537) (44.6407, -39.3669) knots 0 0 0 0 0.065421 0.128708 0.190236 0.250724 0.310637 0.370766 0.431615 0.493523 0.555883 0.617342 0.678668 0.740711 0.802985 0.866803 0.932347 1 1 1 1
  line L69 (44.6407, -39.3669) -> (44.524, -39.3669)
  spline S31 degree 3 poles (44.524, -39.3669) (44.5212, -39.3545) (44.5157, -39.3307) (44.5036, -39.2972) (44.4887, -39.2674) (44.4711, -39.2408) (44.4501, -39.2176) (44.4262, -39.1969) (44.3993, -39.1783) (44.3694, -39.1628) (44.3379, -39.1495) (44.305, -39.1407) (44.2714, -39.1345) (44.2487, -39.1339) (44.2373, -39.1336) knots 0 0 0 0 0.094687 0.181994 0.264377 0.34218 0.418618 0.496509 0.577369 0.661511 0.746733 0.831258 0.915206 1 1 1 1
  spline S32 degree 3 poles (44.2373, -39.1336) (44.2262, -39.1339) (44.2043, -39.1345) (44.172, -39.1391) (44.1409, -39.1462) (44.1112, -39.1569) (44.0824, -39.1698) (44.0552, -39.1864) (44.0289, -39.2055) (44.0042, -39.2274) (43.9816, -39.2516) (43.9616, -39.2774) (43.945, -39.3049) (43.931, -39.3337) (43.9204, -39.364) (43.9128, -39.3958) (43.9083, -39.429) (43.9077, -39.4517) (43.9074, -39.4633) knots 0 0 0 0 0.064207 0.126425 0.18768 0.248216 0.308305 0.369661 0.431699 0.495947 0.559758 0.622295 0.683911 0.745092 0.80674 0.869087 0.93329 1 1 1 1
  spline S33 degree 3 poles (43.9074, -39.4633) (43.9076, -39.4737) (43.9081, -39.4941) (43.912, -39.524) (43.9188, -39.5522) (43.9283, -39.579) (43.9403, -39.6043) (43.9549, -39.6283) (43.9725, -39.6504) (43.9926, -39.6709) (44.0146, -39.6898) (44.0389, -39.7059) (44.065, -39.7194) (44.0926, -39.7311) (44.1223, -39.7395) (44.1535, -39.7458) (44.1866, -39.7495) (44.2093, -39.75) (44.2209, -39.7502) knots 0 0 0 0 0.065351 0.127916 0.18836 0.247216 0.30563 0.36377 0.422661 0.482687 0.5433 0.604118 0.664965 0.727413 0.791468 0.858055 0.927037 1 1 1 1
  spline S34 degree 3 poles (44.2209, -39.7502) (44.231, -39.75) (44.2518, -39.7496) (44.2837, -39.7463) (44.3173, -39.741) (44.3523, -39.7337) (44.3889, -39.7242) (44.4271, -39.7128) (44.4668, -39.6992) (44.4936, -39.6889) (44.5074, -39.6836) knots 0 0 0 0 0.102203 0.211023 0.3251 0.446502 0.573788 0.708901 0.850358 1 1 1 1
  point P0 (22, -80)
  point P1 (32.8574, -36.7836)
  constraints: 140 end point, 30 point on circle, 17 centre point, 72 other
extrude "Выдавливание13" cut sketch "Эскиз14" against normal blind 10 contours A15 | A16
move faces "Перенос1" translate (0, 0, 3) faces at (21.836, 37.9918, 62.5)
